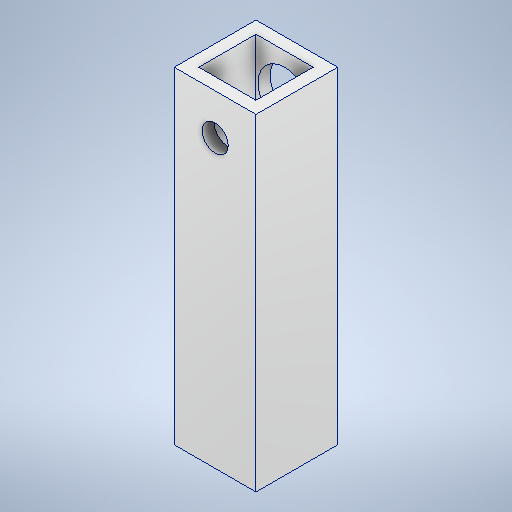
# Autodesk Inventor part: y_standoff
Saved by Autodesk Inventor 2025 (Build 290162000, 162)
## iProperties
Created: 2024-04-25
Part Number: y_standoff
Material: Hliník 6061
Document SubType Name: Modeling
Designer: rader
Density: 2.7 g/cm^3
Appearance: Hliník – plochý
Author: rader
Autodesk Inventor part; units mm, degrees
ref_plane "YZ Plane" through (0, 0, 0) normal (1, 0, 0) x (0, 1, 0)
ref_plane "XZ Plane" through (0, 0, 0) normal (0, 1, 0) x (-1, 0, 0)
ref_plane "XY Plane" through (0, 0, 0) normal (0, 0, 1) x (1, 0, 0)
sketch "Náčrt1" plane through (0, 0, 0) normal (0, 0, 1) x (1, 0, 0)
  line L0 (0, 7) -> (0, -7) projected
  line L1 (-7, 0) -> (7, 0) projected
  line L2 (-3.5, 3.5) -> (3.5, 3.5)
  line L3 (3.5, 3.5) -> (3.5, -3.5)
  line L4 (3.5, -3.5) -> (-3.5, -3.5)
  line L5 (-3.5, -3.5) -> (-3.5, 3.5)
  line L6 (-5, 5) -> (5, 5)
  line L7 (5, 5) -> (5, -5)
  line L8 (5, -5) -> (-5, -5)
  line L9 (-5, -5) -> (-5, 5)
  point P0 (0, 0)
  dimension "d1" = 10
  dimension "d2" = 10
  dimension "d3" = 1.5
  dimension "d4" = 1.5
  dimension "d5" = 1.5
  dimension "d6" = 1.5
  constraints: 16 end point, 4 parallel, 2 horizontal, 2 perpendicular, 2 other
  measures "d1" distance of L6.start L6.end
  measures "d2" distance of L6.end L7.end
  measures "d3" distance between parallel lines of L7 L3
  measures "d4" distance between parallel lines of L9 L5
  measures "d5" distance between parallel lines of L6 L2
  measures "d6" distance between parallel lines of L8 L4
extrude "Vysunutí1" add sketch "Náčrt1" along normal mid plane 40 contours L6 L7 L1 L3 L2 L0 | L0 L2 L5 L1 L9 L6 | L1 L5 L4 L0 L8 L9 | L7 L8 L0 L4 L3 L1
sketch "Náčrt2" plane through (-5, 5, 20) normal (0, 1, 0) x (1, 0, 0)
  line L0 (12, 20) -> (-2, 20) projected
  line L1 (5, 48) -> (5, -8) projected
  line L2 (10, 0) -> (0, 0) projected
  line L3 (0, 40) -> (0, 0) projected
  point P0 (5, 20)
  point P1 (5, 5)
  dimension "d10" = 5
  dimension "d11" = 5
  measures "d10" distance from line of L3 point (5, 5)
  measures "d11" distance from line of L2 point (5, 5)
hole "Díra1" at (0, 5, 15) direction (0, -1, 0) diameter 3.2 end through all counterbore diameter 6.5 counterbore depth 2
sketch "Náčrt3" plane through (-5, 5, 20) normal (0, 1, 0) x (1, 0, 0)
  line L0 (0, 40) -> (0, 0) projected
  line L1 (0, 40) -> (10, 40) projected
  point P0 (5, 20)
  point P1 (5, 34)
  point P2 (5, 22)
  dimension "d19" = 5
  dimension "d20" = 5
  dimension "d21" = 12
  dimension "d22" = 6
  measures "d19" distance from line of L0 point (5, 34)
  measures "d20" distance from line of L0 point (5, 22)
  measures "d21" distance of point (5, 34) point (5, 22)
  measures "d22" distance from line of L1 point (5, 34)
hole "Díra2" at (0, 5, -14) at (0, 5, -2) direction (0, -1, 0) diameter 2.459 depth 1.5 thread size "M3x0.5" class "6H" standard "ISO Metric profile"
